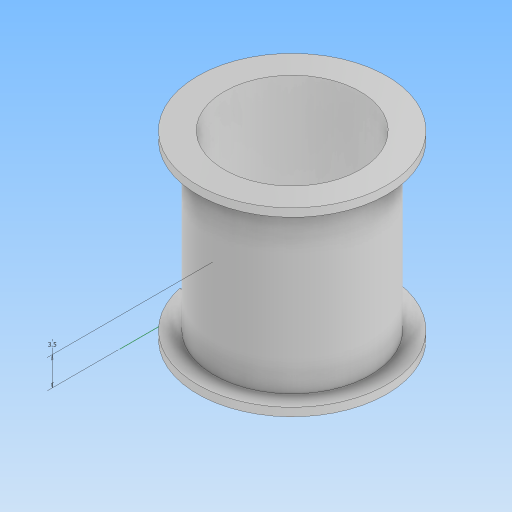
# Autodesk Inventor part: motor JS2622 jsumo
Saved by Autodesk Inventor 2023 (Build 270158000, 158)
## iProperties
Created: 2023-09-08
Part Number: motor JS2622 jsumo
Material: Generic
Document SubType Name: Modeling
Designer: MenMe
Density: 1 g/cm^3
Appearance: Default
Author: MenMe
Autodesk Inventor part; units mm, degrees
ref_plane "XZ Plane" through (0, 0, 0) normal (0, 1, 0) x (-1, 0, 0)
ref_plane "XY Plane" through (0, 0, 0) normal (0, 0, 1) x (1, 0, 0)
sketch "Sketch1" plane through (0, 0, 0) normal (0, 0, 1) x (1, 0, 0)
  line L0 (0, 0) -> (0, 22)
  line L1 (0, 22) -> (11.5, 22)
  line L2 (11.5, 22) -> (11.5, 21)
  line L3 (11.5, 21) -> (9.5, 21)
  line L4 (9.5, 21) -> (9.5, 1)
  line L5 (9.5, 1) -> (11.5, 1)
  line L6 (11.5, 1) -> (11.5, 0)
  line L7 (11.5, 0) -> (0, 0)
  point P0 (5.75, 0)
  dimension "d0" = 22
  dimension "d1" = 20
  dimension "d2" = 1
  dimension "d3" = 23
  dimension "d4" = 19
  constraints: 16 end point, 6 perpendicular, 2 point on line, 1 midpoint, 1 vertical
  measures "d0" distance from line of point (5.75, 0) L1
  measures "d1" distance of L3.end L4.end
  measures "d2" distance of L5.end L6.end
  measures "d3" diameter of L1.end L0
  measures "d4" diameter of L4 L0
revolve "Revolution1" add sketch "Sketch1" angle 360 about axis through (0, 0, 0) along (0, 1, 0)
sketch "Sketch3" plane through (0, 22, 0) normal (0, 1, 0) x (1, 0, 0)
  circle A0 centre (0, 0) radius 8.25
  dimension "d6" = 16.5
  constraints: 1 centre point, 1 coincident
  measures "d6" diameter of A0
extrude "Extrusion1" cut sketch "Sketch3" against normal blind 16
sketch "Sketch4" plane through (0, 0, 0) normal (0, -1, 0) x (1, 0, 0)
  circle A0 centre (0, 0) radius 1.5
  dimension "d9" = 3
  constraints: 1 centre point, 1 coincident
  measures "d9" diameter of A0
extrude "Extrusion2" cut sketch "Sketch4" against normal through all
ref_plane "Work Plane1" through (-9.5, 11, 0) normal (1, 0, 0) x (0, 1, 0)
sketch "Sketch7" plane through (-9.5, 11, 0) normal (1, 0, 0) x (0, 1, 0)
  line L0 (-11, -11.5) -> (-11, 11.5) projected
  point P0 (-11, 0)
  point P1 (-7.5, 0)
  point P2 (-11, 0)
  dimension "d42" = 3.5
  constraints: 1 horizontal alignment, 1 midpoint
  measures "d42" distance from line of point (-7.5, 0) L0
hole "Hole2" at (-9.5, 3.5, 0) direction (-1, 0, 0) diameter 7 end through all
sketch "Sketch8" plane through (-11.5, 0, 0) normal (0, -1, 0) x (1, 0, 0)
  line L0 (6.5, -2.825) -> (9, -2.825)
  line L1 (9, -2.825) -> (9, 2.825)
  line L2 (9, 2.825) -> (6.5, 2.825)
  line L3 (6.5, 2.825) -> (6.5, -2.825)
  circle A0 centre (11.5, 0) radius 9.5 projected
  point P0 (2.235, 2.1)
  point P1 (2.235, -2.1)
  dimension "d58" = 2.5
  dimension "d60" = 2.825
  dimension "d61" = 5.65
  dimension "d62" = 2.5
  constraints: 8 end point, 2 parallel, 1 horizontal, 1 perpendicular
  measures "d58" distance from line of point (11.5, 0) L1
  measures "d60" distance from line of L2 point (11.5, 0)
  measures "d61" distance between parallel lines of L0 L2
  measures "d62" distance of L1.end L2.end
extrude "Extrusion6" cut sketch "Sketch8" along normal through all both and the other way through all contours L3 L2 L1 L0
ref_plane "Work Plane3" through (-8.5, 11, 0) normal (1, 0, 0) x (0, 1, 0)
sketch "Sketch9" plane through (-8.5, 11, 0) normal (1, 0, 0) x (0, 1, 0)
  point P0 (-11, 0)
  point P1 (-7.5, 0)
hole "Hole3" at (-8.5, 3.5, 0) direction (-1, 0, 0) diameter 7 end through all
hole "Hole4" at (-8.5, 3.5, 0) direction (1, 0, 0) diameter 3.5 depth 8.25 countersink diameter 7 countersink angle 90
body "Solid1"
